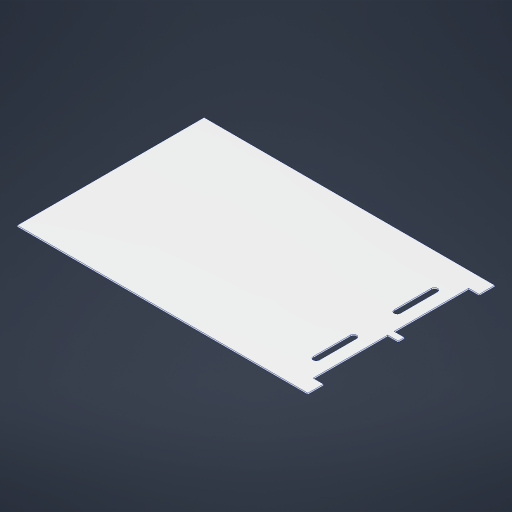
# Autodesk Inventor part: EBox Door
Saved by Autodesk Inventor 2023 (Build 270158000, 158)
## iProperties
Created: 2023-01-27
Part Number: EBox Door
Material: Aluminum 6061
Document SubType Name: Modeling
Designer: Nebil
Density: 2.7 g/cm^3
Appearance: Aluminum - Flat
Author: Nebil
Autodesk Inventor part; units mm, degrees
ref_plane "YZ Plane" through (0, 0, 0) normal (1, 0, 0) x (0, 1, 0)
ref_plane "XZ Plane" through (0, 0, 0) normal (0, 1, 0) x (-1, 0, 0)
ref_plane "XY Plane" through (0, 0, 0) normal (0, 0, 1) x (1, 0, 0)
sketch "Sketch1" plane through (0, 0, 0) normal (0, 1, 0) x (-1, 0, 0)
  line L0 (-177.8, 114.3) -> (177.8, 114.3)
  line L1 (177.8, 114.3) -> (177.8, -114.3)
  line L2 (177.8, -114.3) -> (-177.8, -114.3)
  line L3 (-177.8, -114.3) -> (-177.8, 114.3)
  line L4 (-177.8, 114.3) -> (177.8, -114.3) construction
  line L5 (177.8, 114.3) -> (-177.8, -114.3) construction
  line L6 (-165.1, 95.25) -> (-177.8, 95.25)
  line L7 (-177.8, 95.25) -> (-177.8, 3.81)
  line L8 (-177.8, 3.81) -> (-165.1, 3.81)
  line L9 (-165.1, 3.81) -> (-165.1, 95.25)
  line L10 (-165.1, -3.81) -> (-177.8, -3.81)
  line L11 (-177.8, -3.81) -> (-177.8, -95.25)
  line L12 (-177.8, -95.25) -> (-165.1, -95.25)
  line L13 (-165.1, -95.25) -> (-165.1, -3.81)
  line L14 (-146.05, 72.39) -> (-146.05, 26.67) construction
  line L15 (-149.86, 72.39) -> (-149.86, 26.67)
  line L16 (-142.24, 26.67) -> (-142.24, 72.39)
  arc A0 (-142.24, 72.39) -> (-149.86, 72.39) centre (-146.05, 72.39) ccw
  arc A1 (-149.86, 26.67) -> (-142.24, 26.67) centre (-146.05, 26.67) ccw
  line L17 (-146.05, -26.67) -> (-146.05, -72.39) construction
  line L18 (-149.86, -26.67) -> (-149.86, -72.39)
  line L19 (-142.24, -72.39) -> (-142.24, -26.67)
  arc A2 (-142.24, -26.67) -> (-149.86, -26.67) centre (-146.05, -26.67) ccw
  arc A3 (-149.86, -72.39) -> (-142.24, -72.39) centre (-146.05, -72.39) ccw
  point P0 (0, 0)
  point P1 (-146.05, 49.53)
  point P2 (-146.05, -49.53)
  point P3 (-177.8, 3.81)
  dimension "d0" = 355.6
  dimension "d1" = 228.6
  dimension "d2" = 12.7
  dimension "d3" = 91.44
  dimension "d4" = 91.44
  dimension "d5" = 12.7
  dimension "d6" = 19.05
  dimension "d7" = 19.05
  dimension "d8" = 45.72
  dimension "d9" = 7.62
  dimension "d10" = 45.72
  dimension "d11" = 7.62
  dimension "d12" = 41.91
  dimension "d13" = 19.05
  dimension "d14" = 19.05
  dimension "d15" = 41.91
  constraints: 44 end point, 9 parallel, 8 point on circle, 8 tangent, 4 centre point, 4 midpoint, 3 horizontal, 3 perpendicular, 1 collinear, 1 point on line, 1 vertical
  measures "d0" distance of L1.end L2.end
  measures "d1" distance of L0.end L1.end
  measures "d2" distance of L11.end L12.end
  measures "d3" distance of L12.end L10.start
  measures "d4" distance of L8.end L6.start
  measures "d5" distance of L7.end L8.end
  measures "d6" distance between parallel lines of L2 L12
  measures "d7" distance between parallel lines of L0 L6
  measures "d8" distance of L14.start L14.end
  measures "d9" diameter of A1
  measures "d10" distance of L17.start L17.end
  measures "d11" diameter of A3
  measures "d12" distance from line of L0 L14.start
  measures "d13" distance between parallel lines of L14 L9
  measures "d14" distance between parallel lines of L13 L17
  measures "d15" distance from line of L17.end L2
extrude "Extrusion1" add sketch "Sketch1" along normal blind 1.5875 contours L0 L1 L2 L3 L12 L13 L10 L8 L9 L6
body "Solid1"
